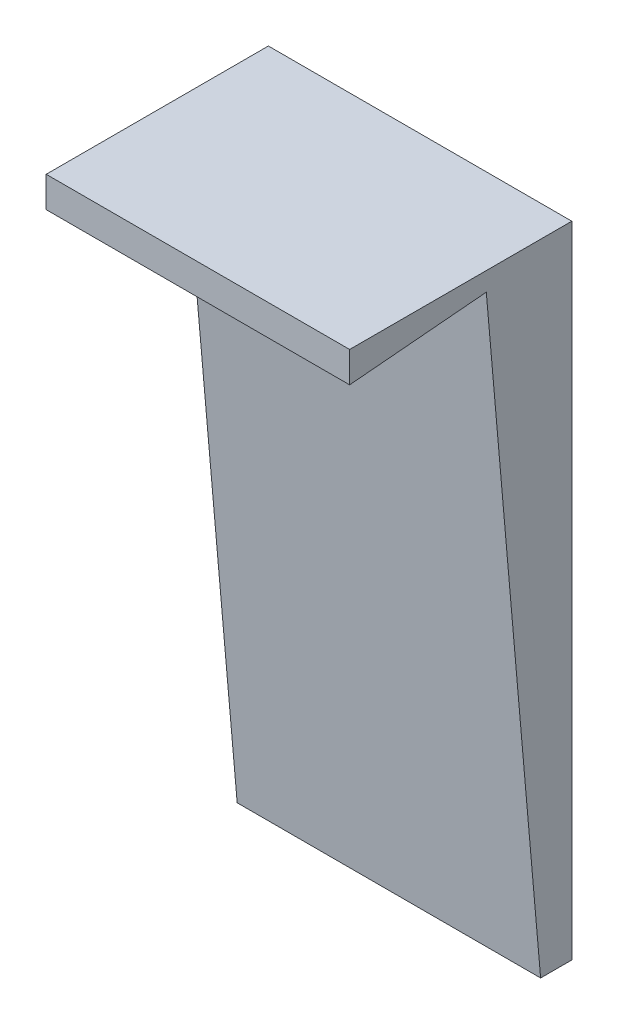
# Autodesk Inventor part: stand
Saved by Autodesk Inventor 2023 (Build 270158000, 158)
## iProperties
Created: 2023-02-16
Part Number: stand
Material: Generic
Document SubType Name: Modeling
Designer: shrey
Density: 1 g/cm^3
Appearance: Default
Author: shrey
Autodesk Inventor part; units mm, degrees
ref_plane "YZ Plane" through (0, 0, 0) normal (1, 0, 0) x (0, 1, 0)
ref_plane "XZ Plane" through (0, 0, 0) normal (0, 1, 0) x (-1, 0, 0)
ref_plane "XY Plane" through (0, 0, 0) normal (0, 0, 1) x (1, 0, 0)
sketch "Sketch1" plane through (0, 0, 0) normal (1, 0, 0) x (0, 1, 0)
  line L0 (0, 21.9163) -> (-204, 21.9163)
  line L1 (-204, 21.9163) -> (-204, -13.7156)
  line L2 (-204, -13.7156) -> (0, -13.7156)
  line L3 (0, -13.7156) -> (0, 21.9163)
  line L4 (-4.9174, 21.9163) -> (-3, 0)
  line L5 (-3, 0) -> (-102.6195, -8.7156)
  line L6 (-102.6195, -8.7156) -> (-102.6195, -13.7156)
  line L7 (-102.6195, -13.7156) -> (0, -13.7156)
  point P0 (0, 0)
  dimension "d0" = 204
  dimension "d2" = 22
  dimension "d3" = 85
  dimension "d5" = 3
  dimension "d6" = 100
  dimension "d7" = 5
  constraints: 16 end point, 3 parallel, 2 perpendicular, 2 point on line, 1 collinear, 1 horizontal, 1 horizontal alignment
  measures "d0" distance of L1.end L2.end
  measures "d2" distance of L4.start L4.end
  measures "d3" angle of L4 L0
  measures "d5" distance from line of L3 L4.end
  measures "d6" distance of L4.end L5.end
  measures "d7" distance of L5.end L6.end
extrude "Extrusion1" add sketch "Sketch1" along normal mid plane 48.6667 contours L3 L2 L6 L5 L4 L0
body "Solid1"
